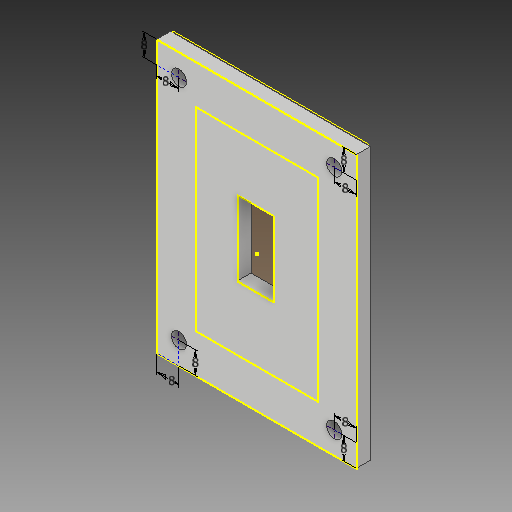
# Autodesk Inventor part: Pieza6
Saved by Autodesk Inventor 2017 (Build 210142000, 142)
## iProperties
Part Number: Pieza6
Material: Genérico
Document SubType Name: Modeling
Designer: user
Density: 1 g/cm^3
Appearance: Valor por defecto
Author: user
Autodesk Inventor part; units mm, degrees
ref_plane "YZ Plane" through (0, 0, 0) normal (1, 0, 0) x (0, 1, 0)
ref_plane "XZ Plane" through (0, 0, 0) normal (0, 1, 0) x (-1, 0, 0)
ref_plane "XY Plane" through (0, 0, 0) normal (0, 0, 1) x (1, 0, 0)
ref_plane "Plano de trabajo1" through (0, 0, 0) normal (0, 0, 1) x (1, 0, 0)
sketch "Boceto1" plane through (0, 0, 0) normal (0, 0, 1) x (1, 0, 0)
  line L0 (-13, -13) -> (-13, 16) projected
  line L1 (-13, 16) -> (16, 16) projected
  line L2 (16, 16) -> (16, -13) projected
  line L3 (16, -13) -> (-13, -13) projected
  line L4 (36, 49) -> (-36, 49) projected
  line L5 (-36, 49) -> (-36, -49) projected
  line L6 (-36, -49) -> (36, -49) projected
  line L7 (36, -49) -> (36, 49) projected
  line L8 (-36, -49) -> (36, -49)
  line L9 (36, -49) -> (36, 49)
  line L10 (36, 49) -> (-36, 49)
  line L11 (-36, 49) -> (-36, -49)
  line L12 (6, 15) -> (-7, 15) projected
  line L13 (-7, 15) -> (-7, -12) projected
  line L14 (-7, -12) -> (6, -12) projected
  line L15 (6, -12) -> (6, 15) projected
  line L16 (-7, -12) -> (6, -12)
  line L17 (6, -12) -> (6, 15)
  line L18 (6, 15) -> (-7, 15)
  line L19 (-7, 15) -> (-7, -12)
  circle A0 centre (28, -41) radius 2.75 projected
  circle A1 centre (-28, 41) radius 2.75 projected
  circle A2 centre (28, 41) radius 2.75 projected
  circle A3 centre (-28, -41) radius 2.75 projected
  point P0 (0, 0)
  constraints: 16 end point, 4 parallel, 2 horizontal, 2 perpendicular
extrude "Extrusión1" add sketch "Boceto1" along normal blind 5 contours L0 L1 L2 L3 | L7 L6 L5 L4 | A0 | A1 | A2 | A3
sketch "Boceto3" plane through (0, 0, 5) normal (0, 0, 1) x (1, 0, 0)
  line L0 (6, 15) -> (6, -12) projected
  line L1 (6, -12) -> (-7, -12) projected
  line L2 (-7, -12) -> (-7, 15) projected
  line L3 (-7, 15) -> (6, 15) projected
  line L4 (36, 49) -> (-36, 49) projected
  line L5 (-36, 49) -> (-36, -49) projected
  line L6 (-36, -49) -> (36, -49) projected
  line L7 (36, -49) -> (36, 49) projected
  line L8 (-36, -49) -> (36, -49) construction
  line L9 (-36, -49) -> (-28, -49) construction
  line L10 (-28, -49) -> (-28, -41) construction
  line L11 (-22, -35) -> (22, -35) projected
  line L12 (-22, 35) -> (-22, -35) projected
  line L13 (22, 35) -> (-22, 35) projected
  line L14 (22, -35) -> (22, 35) projected
  line L15 (36, -49) -> (36, -41) construction
  line L16 (36, -49) -> (36, 49) construction
  line L17 (36, -41) -> (28, -41) construction
  line L18 (36, 49) -> (36, 41) construction
  line L19 (36, 41) -> (28, 41) construction
  line L20 (-36, 49) -> (-36, -49) construction
  line L21 (-36, 49) -> (-36, 41) construction
  line L22 (-36, 41) -> (-28, 41) construction
  point P0 (0, 0)
  dimension "d2" = 8
  dimension "d3" = 8
  dimension "d4" = 8
  dimension "d5" = 8
  dimension "d6" = 8
  dimension "d7" = 8
  dimension "d8" = 8
  dimension "d9" = 8
  constraints: 16 end point, 4 coincident, 4 point on line, 3 perpendicular, 1 horizontal
  measures "d2" distance of L5.end L9.end
  measures "d3" distance of L9.end L10.end
  measures "d4" distance of L6.end L15.end
  measures "d5" distance of L15.end L17.end
  measures "d6" distance of L4.start L18.end
  measures "d7" distance of L18.end L19.end
  measures "d8" distance of L4.end L21.end
  measures "d9" distance of L21.end L22.end
sketch "Boceto4" plane through (0, 0, 5) normal (0, 0, 1) x (1, 0, 0)
  point P0 (-28, 41)
  point P1 (28, 41)
  point P2 (28, -41)
  point P3 (-28, -41)
hole "Agujero1" at (-28, 41, 5) at (28, 41, 5) at (28, -41, 5) at (-28, -41, 5) direction (0, 0, -1) diameter 5.5 depth 5
sketch "Boceto5" plane through (0, 0, 5) normal (0, 0, 1) x (1, 0, 0)
  point P0 (0, 0)
